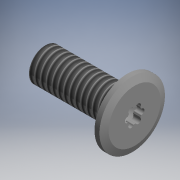
# Autodesk Inventor part: CBSTSE4-10
Saved by Autodesk Inventor 2017.3 (Build 213256000, 256)
## iProperties
Part Number: CBSTSE4-10
Material: Generic
Catalog Web Link: www.cadenas.de
Description: CBSSE, CBSKE, CBSTSE-Ultra Low Head Cap Screws
Vendor: MISUMI
Document SubType Name: Modeling
Designer: partserver
Manufacturer: MISUMI
Mass: 0.164535 g
Surface Area: 2.50032 cm^2
Volume: 0.164535 cm^3
Density: 1 g/cm^3
Appearance: PSOLRGB-175-175-175
Category: PARTsolutions
Company: MISUMI
Title: CBSTSE4-10
Author: Cadenas PARTsolutions
Comments: Ultra Low Head Cap Screws
PSOL_IDENT_0: {$CADENAS_DATA\23d-libs\misumi\metric\27_screws_nuts\cbsse.prj},183 {VTYP=3D},{NB=CBSTSE4-10},{LINA=
PSOL_IDENT_1: CBSTSE4-10},{NN=CBSSE, CBSKE, CBSTSE},{DATE=30.06.2021 13:09:26},{GEOMDATE=06.03.2020 06:08:05},{VER
PSOL_IDENT_2: SION=},{LINEID=40},{WBVAR=MAT,ST,L},{WBNUMERIC=L}  {NB=CBSTSE4-10},{LINA=CBSTSE4-10},{KT=DUMMY},{PN=
PSOL_IDENT_3: CBSTSE4-10},{TYPE=CBSTSE},{MAT=2},{MATA=  '1','Cold Forged Carbon Steel Wire SWCH12~18A','2','304 St
PSOL_IDENT_4: ainless Steel'    },{HARD=-},{ST=3},{STA=  '3','-'    },{M=4},{M1=4.0},{L=10},{L0=5,6,8,10,12,16,20,
PSOL_IDENT_5: 25},{MP=M4x0.7},{A=8},{B=1.75},{E=0.9},{C=2.40},{TT=0.90},{RR=0.5},{P=0.70}
NB: CBSTSE4-10
NN: CBSSE, CBSKE, CBSTSE
NT: Ultra Low Head Cap Screws
NBSYN: $PN.
LINA: CBSTSE4-10
CATALOG: Misumi
PN: CBSTSE4-10
TYPE: CBSTSE
MAT: 304 Stainless Steel
HARD: -
ST: -
M: 4
L: 10
MP: M4x0.7
A: 8
B: 1.75
E: 0.9
TT: 0.9
RR: 0.5
SUPPLIER: MISUMI
ARTICLENO: CBSTSE4-10
BOMINFO: CBSTSE4-10
CREATOR: CADENAS GmbH
Autodesk Inventor part; units mm, degrees
ref_plane "YZ Plane" through (0, 0, 0) normal (1, 0, 0) x (0, 1, 0)
ref_plane "XZ Plane" through (0, 0, 0) normal (0, 1, 0) x (-1, 0, 0)
ref_plane "XY Plane" through (0, 0, 0) normal (0, 0, 1) x (1, 0, 0)
sketch "Sketch_1" plane through (0, 0, 0) normal (0, 0, 1) x (1, 0, 0)
  line L0 (10, 0) -> (-0.9, 0)
  line L1 (-0.9, 0) -> (-0.9, 3.1758)
  line L2 (-0.9, 3.1758) -> (-0.6, 4)
  line L3 (-0.6, 4) -> (0, 4)
  line L4 (0, 4) -> (0, 2.5)
  arc A0 (0, 2.5) -> (0.5, 2) centre (0.5, 2.5) ccw
  line L5 (0.5, 2) -> (10, 2)
  line L6 (10, 2) -> (10, 0)
  line L7 (10, 0) -> (-0.9, 0)
  constraints: 16 end point, 2 point on circle, 1 centre point
revolve "Revolution1" add sketch "Sketch_1" angle 360 about axis through (10, 0, 0) along (1, 0, 0)
thread "Thread1" size "M4x0.7" class "6g" standard "ISO Metric profile" length 9.3 offset 0.2
sketch "Sketch_5" plane through (0, 0, 0) normal (1, 0, 0) x (0, 0, -1)
  arc A0 (-0.9219, -0.157) -> (-0.5969, -0.7199) centre (-0.7578, -0.4375) ccw
  arc A1 (-0.4913, -0.7241) -> (-0.5969, -0.7199) centre (-0.5474, -0.8068) ccw
  arc A2 (-0.4913, -0.7241) -> (-0.3814, -0.7875) centre (0, 0) ccw
  arc A3 (-0.325, -0.8769) -> (-0.3814, -0.7875) centre (-0.425, -0.8775) ccw
  arc A4 (-0.325, -0.8769) -> (0.325, -0.8769) centre (0, -0.875) ccw
  arc A5 (0.3814, -0.7875) -> (0.325, -0.8769) centre (0.425, -0.8775) ccw
  arc A6 (0.3814, -0.7875) -> (0.4913, -0.7241) centre (0, 0) ccw
  arc A7 (0.5969, -0.7199) -> (0.4913, -0.7241) centre (0.5474, -0.8068) ccw
  arc A8 (0.5969, -0.7199) -> (0.9219, -0.157) centre (0.7578, -0.4375) ccw
  arc A9 (0.8727, -0.0634) -> (0.9219, -0.157) centre (0.9724, -0.0707) ccw
  arc A10 (0.8727, -0.0634) -> (0.8727, 0.0634) centre (0, 0) ccw
  arc A11 (0.9219, 0.157) -> (0.8727, 0.0634) centre (0.9724, 0.0707) ccw
  arc A12 (0.9219, 0.157) -> (0.5969, 0.7199) centre (0.7578, 0.4375) ccw
  arc A13 (0.4913, 0.7241) -> (0.5969, 0.7199) centre (0.5474, 0.8068) ccw
  arc A14 (0.4913, 0.7241) -> (0.3814, 0.7875) centre (0, 0) ccw
  arc A15 (0.325, 0.8769) -> (0.3814, 0.7875) centre (0.425, 0.8775) ccw
  arc A16 (0.325, 0.8769) -> (-0.325, 0.8769) centre (0, 0.875) ccw
  arc A17 (-0.3814, 0.7875) -> (-0.325, 0.8769) centre (-0.425, 0.8775) ccw
  arc A18 (-0.3814, 0.7875) -> (-0.4913, 0.7241) centre (0, 0) ccw
  arc A19 (-0.5969, 0.7199) -> (-0.4913, 0.7241) centre (-0.5474, 0.8068) ccw
  arc A20 (-0.5969, 0.7199) -> (-0.9219, 0.157) centre (-0.7578, 0.4375) ccw
  arc A21 (-0.8727, 0.0634) -> (-0.9219, 0.157) centre (-0.9724, 0.0707) ccw
  arc A22 (-0.8727, 0.0634) -> (-0.8727, -0.0634) centre (0, 0) ccw
  arc A23 (-0.9219, -0.157) -> (-0.8727, -0.0634) centre (-0.9724, -0.0707) ccw
  constraints: 48 point on circle, 24 centre point
extrude "Extrusion1" cut sketch "Sketch_5" against normal blind 0.9
sketch "Sketch_2" plane through (0, 0, 0) normal (0, 0, 1) x (1, 0, 0)
  line L0 (0.6928, 0) -> (0, 0)
  line L1 (0, 0) -> (0, 1.2)
  line L2 (0, 1.2) -> (0.6928, 0)
  line L3 (0.6928, 0) -> (0, 0)
  constraints: 8 end point
revolve "Revolution2" cut sketch "Sketch_2" angle 360 about axis through (0.6928, 0, 0) along (1, 0, 0)
body "Solid1"
